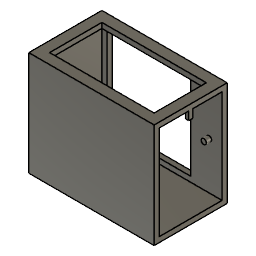
Case (Autodesk Fusion 360 design; units mm, degrees)
part number: 2026-05-08-17-20-08-831
Autodesk Fusion 360 part; units mm, degrees
sketch "case" plane through (0, 0, 0) normal (1, 0, 0) x (0, 1, 0)
  line L0 (0, 0) -> (70, 0)
  line L1 (70, 0) -> (70, 100)
  line L2 (70, 100) -> (0, 100)
  line L3 (0, 100) -> (0, 0)
  line L4 (65, 95) -> (5, 95)
  line L5 (5, 95) -> (5, 5)
  line L6 (5, 5) -> (65, 5)
  line L7 (65, 5) -> (65, 95)
  line L8 (33, 95) -> (33, 87)
  line L9 (33, 87) -> (37, 87)
  line L10 (37, 87) -> (37, 95)
  dimension "d23" = 70
  dimension "d24" = 100
  dimension "d25" = -5
  dimension "d26" = 8
  dimension "d27" = 4
  dimension "d28" = 28
  constraint coincident L0.start L3.end
  constraint horizontal L0
  constraint perpendicular L0 L1
  constraint perpendicular L1 L2
  constraint perpendicular L0 L3
  constraint coincident L4 L8.start
  constraint perpendicular L4 L8
  constraint perpendicular L8 L9
  constraint perpendicular L4 L10
  constraint coincident L4 L10.end
  measures "d23" distance of L0.start L0.end
  measures "d24" distance of L0.end L1.end
  measures "d26" distance of L8.start L8.end
  measures "d27" distance of L8.end L9.end
  measures "d28" distance of L5 L8
extrude "Extrude4" add sketch "case" along normal blind 5 contours L0 L1 L2 L3 | L4 L5 L6 L7 L8 L9 L10 | L4 L8 L9 L10
extrude "Extrude5" add sketch "case" along normal blind 120
extrude "Extrude6" add sketch "case" against normal blind 3 from surface at 120 contours L4 L8 L9 L10
sketch "side" plane through (0, 0, 0) normal (0, 1, 0) x (1, 0, 0)
  line L0 (120, -100) -> (120, 0)
  line L1 (0, -100) -> (120, -100)
  line L2 (0, 0) -> (120, 0)
  line L3 (0, -100) -> (0, 0)
  circle A0 centre (107.5, -50) radius 2.5
  circle A1 centre (75, -50) radius 2.5
  circle A2 centre (42.5, -50) radius 2.5
  circle A3 centre (42.5, -50) radius 1.6
  line L4 (10, -10) -> (90, -10)
  line L5 (90, -10) -> (90, -90)
  line L6 (90, -90) -> (10, -90)
  line L7 (10, -90) -> (10, -10)
  circle A4 centre (42.5, -50) radius 12.5 construction
  circle A5 centre (75, -50) radius 20 construction
  circle A6 centre (50, -34.7439) radius 1.4
  circle A7 centre (50, -34.7439) radius 2.5
  line L8 (55, -50) -> (50, -34.7439) construction
  line L9 (48.5, -39.7439) -> (60.5, -39.7439) construction
  circle A8 centre (54.5, -39.7439) radius 1.75
  circle A9 centre (23.5, -50) radius 1.75
  circle A10 centre (17.6, -57.532) radius 1.4
  circle A11 centre (17.6, -57.532) radius 2.5
  dimension "d36" = 5
  dimension "d37" = 12.5
  dimension "d38" = 50
  dimension "d45" = 32.5
  dimension "d47" = 50
  dimension "d48" = 5
  dimension "d52" = 32.5
  dimension "d53" = 50
  dimension "d54" = 5
  dimension "d58" = 3.2
  dimension "d66" = 10
  dimension "d67" = 10
  dimension "d68" = 10
  dimension "d91" = 30
  dimension "d92" = 25
  dimension "d93" = 40
  dimension "d94" = 2.8
  dimension "d95" = 5
  dimension "d96" = 17
  dimension "d97" = 40
  dimension "d103" = 5
  dimension "d104" = 3.5
  dimension "d105" = 12
  dimension "d106" = 44.5
  dimension "d114" = 3.5
  dimension "d115" = 50
  dimension "d116" = 19
  dimension "d146" = 2.8
  dimension "d147" = 17.6
  dimension "d148" = 42.468
  dimension "d152" = 5
  constraint concentric A2 A3
  constraint horizontal L4
  constraint perpendicular L4 L5
  constraint perpendicular L5 L6
  constraint perpendicular L4 L7
  constraint concentric A3 A4
  constraint concentric A1 A5
  constraint concentric A6 A7
  constraint coincident A4 L8.start
  constraint coincident A5 L8.start
  constraint coincident A6.centre A7.centre
  constraint horizontal L9
  constraint coincident L9 A8.centre
  constraint midpoint L9 A8.centre
  constraint concentric A10 A11
  measures "d36" diameter of A0
  measures "d37" distance of L0 A0.centre
  measures "d38" distance of L1 A0.centre
  measures "d45" distance of A0.centre A1.centre
  measures "d47" distance of L1 A1.centre
  measures "d48" diameter of A1
  measures "d52" horizontal distance of A1.centre A2.centre
  measures "d53" distance of L1 A2.centre
  measures "d54" diameter of A2
  measures "d58" diameter of A3
  measures "d66" distance of L1 L6
  measures "d67" distance of L3 L7
  measures "d68" distance of L2 L4
  measures "d91" distance of L0 L5
  measures "d92" diameter of A4
  measures "d93" diameter of A5
  measures "d94" diameter of A6
  measures "d95" diameter of A7
  measures "d96" distance of A2.centre A6.centre
  measures "d97" distance of L7 A6.centre
  measures "d103" distance of A6.centre L9
  measures "d104" diameter of A8
  measures "d105" distance of L9.start L9.end
  measures "d106" distance of L7 A8.centre
  measures "d114" diameter of A9
  measures "d115" distance of L1 A9.centre
  measures "d116" distance of A2.centre A9.centre
  measures "d146" diameter of A10
  measures "d147" distance of L3 A10.centre
  measures "d148" distance of L1 A10.centre
  measures "d152" diameter of A11
extrude "Extrude7" add sketch "side" along normal blind 5 from surface at 5 contours A0 | A1 | A2 | A3
extrude "Extrude8" add sketch "side" against normal blind 5 from surface at 65 contours A0
extrude "Extrude11" add sketch "side" along normal blind 5 from surface at 10 contours A3
extrude "Extrude12" cut sketch "side" along normal up to surface (5 mm away) from surface at 65 contours A1 | A2 | A3 | L4 L5 L6 L7 | A6 | A7 | A8 | A9 | A10 | A11
sketch "top" plane through (0, 0, 100) normal (0, 0, 1) x (-1, 0, 0)
  line L0 (0, -70) -> (0, 0)
  line L1 (0, 0) -> (-120, 0)
  line L2 (-120, 0) -> (-120, -70)
  line L3 (-120, -70) -> (0, -70)
  line L4 (-10, -10) -> (-110, -10)
  line L5 (-110, -10) -> (-110, -60)
  line L6 (-110, -60) -> (-10, -60)
  line L7 (-10, -60) -> (-10, -10)
  dimension "d90" = -10
extrude "Extrude14" add sketch "side" along normal blind 5.5 from surface at 5 contours A6 | A7
extrude "Extrude16" add sketch "side" along normal blind 5.2 contours A6 | A7
extrude "Extrude17" add sketch "side" along normal blind 5 from surface at 10.5 contours A6
extrude "Extrude18" add sketch "side" along normal blind 16 from surface at 5 contours A8 | A9
extrude "Extrude19" cut sketch "top" against normal up to surface (5 mm away) contours L4 L5 L6 L7
sketch "back" plane through (0, 0, 0) normal (-1, 0, 0) x (0, -1, 0)
  line L0 (0, 0) -> (0, 100)
  line L1 (0, 100) -> (-70, 100)
  line L2 (-70, 100) -> (-70, 0)
  line L3 (-70, 0) -> (0, 0)
  line L4 (0, 100) -> (0, 0)
  line L5 (0, 0) -> (-70, 0)
  line L6 (-70, 0) -> (-70, 100)
  line L7 (-70, 100) -> (0, 100)
  line L8 (-21, 57) -> (-9, 57)
  line L9 (-9, 57) -> (-9, 48)
  line L10 (-9, 48) -> (-21, 48)
  line L11 (-21, 48) -> (-21, 57)
  line L12 (-60, 100) -> (-10, 100)
  line L13 (0, 90) -> (0, 10)
  line L14 (-23, 59) -> (-7, 59)
  line L15 (-7, 59) -> (-7, 46)
  line L16 (-7, 46) -> (-23, 46)
  line L17 (-23, 46) -> (-23, 59)
  dimension "d117" = 43
  dimension "d118" = 12
  dimension "d119" = 9
  dimension "d120" = 9
  dimension "d121" = -2
  constraint horizontal L8
  constraint vertical L9
  constraint horizontal L10
  constraint vertical L11
  measures "d117" distance of L8 L12
  measures "d118" distance of L9.end L10.end
  measures "d119" distance of L9 L13
  measures "d120" distance of L8.start L10.end
extrude "Extrude21" cut sketch "back" against normal up to surface (5 mm away) contours L8 L9 L10 L11
extrude "Extrude22" add sketch "side" along normal blind 17 contours A10
extrude "Extrude23" add sketch "side" along normal blind 9.8 contours A10 | A11
equation "d28 = ( d23 + d25 * 2 - d27 ) / 2"
equation "d37 = ( 25 / 2 ) * 1 mm"
equation "d38 = ( 100 / 2 ) * 1 mm"
equation "d45 = ( 25 / 2 ) * 1 mm + 20 mm"
equation "d47 = d38"
equation "d48 = d36"
equation "d52 = d45"
equation "d53 = d47"
equation "d54 = d48"
equation "d114 = d104"
equation "d115 = d53"
equation "d150 = 5 mm + 12 mm"
equation "d153 = 5 mm + 4.8 mm"
named bodies: "case"
